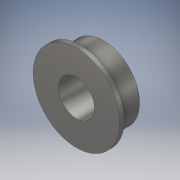
# Autodesk Inventor part: bear_f4_sa_1
Saved by Autodesk Inventor 2019 (Build 230136000, 136)
## iProperties
Created: 2018-12-17
Part Number: bear_f4_sa_1
Material: ステンレス鋼
Document SubType Name: Modeling
Designer: shun
Density: 8 g/cm^3
Appearance: 半つや出し
Author: shun
Autodesk Inventor part; units mm, degrees
ref_plane "YZ Plane" through (0, 0, 0) normal (1, 0, 0) x (0, 1, 0)
ref_plane "XZ Plane" through (0, 0, 0) normal (0, 1, 0) x (-1, 0, 0)
ref_plane "XY Plane" through (0, 0, 0) normal (0, 0, 1) x (1, 0, 0)
sketch "スケッチ1" plane through (0, 0, 0) normal (0, 1, 0) x (-1, 0, 0)
  line L0 (0, 0) -> (-2, 0) construction
  line L1 (-2, 0) -> (-4.8, 0)
  line L2 (-4.8, 0) -> (-4.8, -0.5)
  line L3 (-2, 0) -> (-2, -3)
  line L4 (-2, -3) -> (-4, -3)
  line L5 (-4, -3) -> (-4, -0.5)
  line L6 (-4, -0.5) -> (-4.8, -0.5)
  line L7 (0, -3.6) -> (0, 0.6) projected
  dimension "d0" = 2
  dimension "d1" = 2.8
  dimension "d2" = 0.5
  dimension "d3" = 2
  dimension "d4" = 2.5
  constraints: 14 end point, 4 perpendicular, 2 horizontal, 1 vertical
  measures "d0" distance of L0.start L0.end
  measures "d1" distance of L0.end L1.end
  measures "d2" distance of L1.end L2.end
  measures "d3" distance of L3.end L4.end
  measures "d4" distance of L4.end L5.end
revolve "回転1" add sketch "スケッチ1" angle 360 about axis through (0, 0, -10) along (0, 0, 1)
